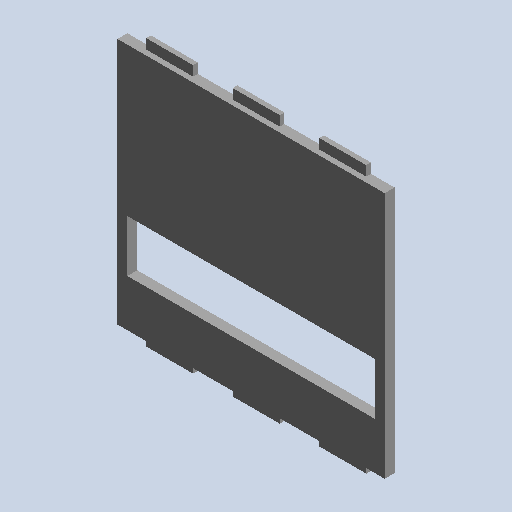
# Autodesk Inventor part: Enclosure_4
Saved by Autodesk Inventor 2026 (Build 300175050, 175E)
## iProperties
Part Number: Enclosure_4
Material: Generic
Document SubType Name: Modeling
Designer: Kartik
Mass: 35.6664 g
Surface Area: 210.352 cm^2
Volume: 35.6664 cm^3
Density: 1 g/cm^3
Appearance: Default
Author: Kartik
Autodesk Inventor part; units mm, degrees
ref_plane "YZ Plane" through (0, 0, 0) normal (1, 0, 0) x (0, 1, 0)
ref_plane "XZ Plane" through (0, 0, 0) normal (0, 1, 0) x (-1, 0, 0)
ref_plane "XY Plane" through (0, 0, 0) normal (0, 0, 1) x (1, 0, 0)
sketch "Sketch1" plane through (0, 0, 0) normal (0, 0, 1) x (1, 0, 0)
  line L0 (-0.0716, 53.5507) -> (107.9284, 53.5507)
  line L1 (107.9284, 53.5507) -> (107.9284, -46.4493)
  line L2 (107.9284, -46.4493) -> (-0.0716, -46.4493)
  line L3 (-0.0716, -46.4493) -> (-0.0716, 53.5507)
  point P0 (0, 0)
  dimension "d0" = 108
  dimension "d1" = 100
  constraints: 8 end point, 2 parallel, 1 horizontal, 1 perpendicular
  measures "d0" distance of L0.start L0.end
  measures "d1" distance of L0.end L1.end
extrude "Extrusion1" add sketch "Sketch1" along normal blind 4
sketch "Sketch2" plane through (-0.0716, 53.5507, 0) normal (0, 1, 0) x (1, 0, 0)
  line L0 (0, 0) -> (108, 0) projected
  line L1 (9.5, 0) -> (28.5, 0)
  line L2 (28.5, 0) -> (28.5, -1.9)
  line L3 (28.5, -1.9) -> (9.5, -1.9)
  line L4 (9.5, -1.9) -> (9.5, 0)
  point P0 (0.0716, 0)
  point P1 (28.5, 0)
  dimension "d4" = 19
  dimension "d5" = 1.9
  dimension "d6" = 9.5
  constraints: 8 end point, 2 parallel, 1 horizontal, 1 perpendicular, 1 point on line
  measures "d4" distance of L2.end L3.end
  measures "d5" distance of L1.end L2.end
  measures "d6" distance from line of L4 L0.start
extrude "Extrusion2" add sketch "Sketch2" along normal blind 4
pattern_linear "Rectangular Pattern1" count 3 spacing 35 along (1, 0, 0) count 2 spacing 104 along (0, -1, 0) of "Extrusion2"
sketch "Sketch3" plane through (0, 0, 4) normal (0, 0, 1) x (1, 0, 0)
  line L0 (3.9284, -6.4493) -> (103.9284, -6.4493)
  line L1 (103.9284, -6.4493) -> (103.9284, -27.4493)
  line L2 (103.9284, -27.4493) -> (3.9284, -27.4493)
  line L3 (3.9284, -27.4493) -> (3.9284, -6.4493)
  line L4 (-0.0716, 53.5507) -> (-0.0716, -46.4493) projected
  line L5 (107.9284, 53.5507) -> (-0.0716, 53.5507) projected
  point P0 (0, 0)
  dimension "d15" = 100
  dimension "d16" = 21
  dimension "d17" = 4
  dimension "d18" = 60
  constraints: 8 end point, 2 parallel, 1 horizontal, 1 perpendicular
  measures "d15" distance of L1.end L2.end
  measures "d16" distance of L0.end L1.end
  measures "d17" distance between parallel lines of L4 L3
  measures "d18" distance between parallel lines of L5 L0
extrude "Extrusion3" cut sketch "Sketch3" against normal blind 4
body "Solid1"
